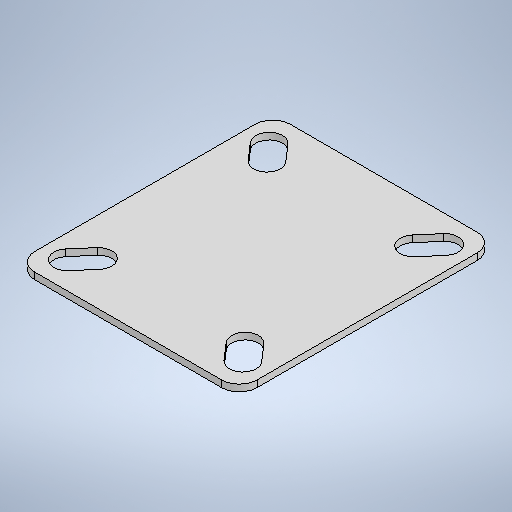
# Autodesk Inventor part: AQUA AISI304 4vv wheel plate 150
Saved by Autodesk Inventor 2025.1 (Build 291241020, 241B)
## iProperties
Created: 2024-11-20
Part Number: AQUA AISI304 4vv wheel plate 150
Material: Stainless Steel
Document SubType Name: Sheet Metal
Designer: user
Mass: 280.619 g
Surface Area: 364.406 cm^2
Volume: 35.0774 cm^3
Density: 8 g/cm^3
Sheet Metal Rule: AISI304 3mm Die 32
Sheet Metal Width: 100.000 mm
Sheet Metal Length: 115.000 mm
Sheet Metal Area: 11500.000 mm^2
Appearance: Default
Flat Pattern Width: 10 cm
Flat Pattern Length: 11.5 cm
Flat Pattern Area: 115 cm^2
Author: user
Autodesk Inventor part; units mm, degrees
ref_plane "YZ Plane" through (0, 0, 0) normal (1, 0, 0) x (0, 1, 0)
ref_plane "XZ Plane" through (0, 0, 0) normal (0, 1, 0) x (-1, 0, 0)
ref_plane "XY Plane" through (0, 0, 0) normal (0, 0, 1) x (1, 0, 0)
sketch "Sketch1" plane through (0, 0, 0) normal (0, 0, 1) x (1, 0, 0)
  line L0 (-50, -57.5) -> (50, -57.5)
  line L1 (50, -57.5) -> (50, 57.5)
  line L2 (50, 57.5) -> (-50, 57.5)
  line L3 (-50, 57.5) -> (-50, -57.5)
  line L4 (-50, -57.5) -> (50, 57.5) construction
  line L5 (50, -57.5) -> (-50, 57.5) construction
  point P0 (0, 0)
  dimension "d0" = 100
  dimension "d1" = 115
  measures "d0" distance of L2.end L1.end
  measures "d1" distance of L1.end L0.end
extrude "Plate1" add sketch "Sketch1" along normal blind 3
sketch "Sketch5" plane through (0, 0, 3) normal (0, 0, 1) x (1, 0, 0)
  line L0 (50, -57.5) -> (-50, -57.5) construction
  line L1 (50, 57.5) -> (50, -57.5) construction
  line L2 (-50, 57.5) -> (50, 57.5) construction
  line L3 (-50, -57.5) -> (-50, 57.5) construction
  line L4 (50, 57.5) -> (-50, 57.5) construction
  line L5 (-50, 57.5) -> (50, -57.5) construction
  line L6 (-39.5011, 45.4263) -> (-32.9394, 37.8803) construction
  line L7 (-44.0288, 41.4892) -> (-37.467, 33.9432)
  line L8 (-28.4117, 41.8173) -> (-34.9735, 49.3634)
  arc A0 (-34.9735, 49.3634) -> (-44.0288, 41.4892) centre (-39.5011, 45.4263) ccw
  arc A1 (-37.467, 33.9432) -> (-28.4117, 41.8173) centre (-32.9394, 37.8803) ccw
  point P0 (0, 0)
  point P1 (-36.2202, 41.6533)
  dimension "d22" = 12
  dimension "d23" = 10
  dimension "d24" = 16
  constraints: 10 end point, 4 point on circle, 4 tangent, 2 centre point, 2 point on line, 1 midpoint, 1 parallel
  measures "d22" diameter of A1
  measures "d23" distance of L6.end L6.start
  measures "d24" distance of L2.start L6.start
extrude "Cut1" cut sketch "Sketch5" against normal blind 3
mirror "Mirror1" about plane through (0, 0, 0) normal (0, 1, 0) of "Cut1"
mirror "Mirror2" about plane through (0, 0, 0) normal (1, 0, 0) of "Cut1", "Mirror1"
fillet "Corner Round1" radius 8 4 edges at (-50, 57.5, 1.5) (50, 57.5, 1.5) (50, -57.5, 1.5) (-50, -57.5, 1.5)
equation "\"d25\" = Thickness"
equation "\"d2\" = Thickness"
equation "\"BendReliefWidth\" = Thickness"
equation "\"BendReliefDepth\" = 0.5 * Thickness"
equation "\"CornerReliefSize\" = 4 * Thickness"
equation "\"MinimumRemnant\" = 2 * Thickness"
equation "\"TransitionRadius\" = BendRadius"
equation "\"JacobiRadiusSize\" = BendRadius"
equation "\"GapSize\" = Thickness"
equation "\"Thickness\" = 3"
equation "\"BendRadius\" = 5"
body "Solid1"
